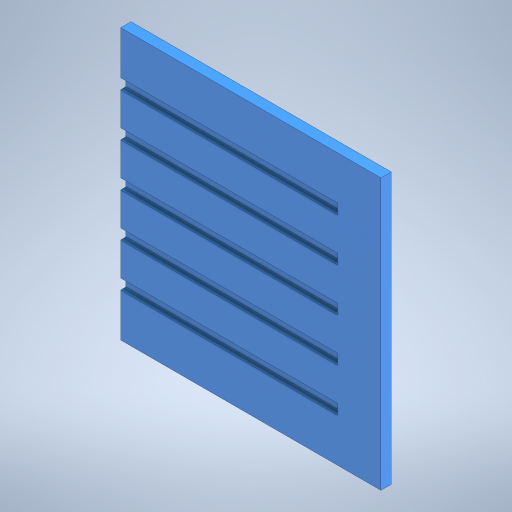
# Autodesk Inventor part: FrntBck Plate
Saved by Autodesk Inventor 2024 (Build 280153000, 153)
## iProperties
Created: 2023-10-03
Part Number: FrntBck Plate
Material: Generic
Document SubType Name: Modeling
Designer: flynf
Density: 1 g/cm^3
Appearance: Cyan
Author: flynf
Autodesk Inventor part; units mm, degrees
ref_plane "YZ Plane" through (0, 0, 0) normal (1, 0, 0) x (0, 1, 0)
ref_plane "XZ Plane" through (0, 0, 0) normal (0, 1, 0) x (-1, 0, 0)
ref_plane "XY Plane" through (0, 0, 0) normal (0, 0, 1) x (1, 0, 0)
sketch "Sketch1" plane through (0, 0, 0) normal (0, 0, 1) x (1, 0, 0)
  line L0 (0, 0) -> (279.4, 0)
  line L1 (279.4, 0) -> (279.4, 279.4)
  line L2 (279.4, 279.4) -> (0, 279.4)
  line L3 (0, 279.4) -> (0, 0)
  dimension "d0" = 279.4
  dimension "d1" = 279.4
  constraints: 8 end point, 2 parallel, 1 horizontal, 1 perpendicular
  measures "d0" distance of L0.end L1.end
  measures "d1" distance of L0.start L0.end
extrude "Extrusion1" add sketch "Sketch1" along normal blind 12.7
sketch "Sketch2" plane through (0, 0, 12.7) normal (0, 0, 1) x (1, 0, 0)
  line L0 (279.4, 0) -> (279.4, 279.4) projected
  line L1 (0, 0) -> (279.4, 0)
  line L2 (279.4, 0) -> (279.4, 12.7)
  line L3 (279.4, 12.7) -> (0, 12.7)
  line L4 (0, 12.7) -> (0, 0)
  line L5 (0, 279.4) -> (0, 0) projected
  line L6 (0, 53.34) -> (279.4, 53.34)
  line L7 (279.4, 53.34) -> (279.4, 66.04)
  line L8 (279.4, 66.04) -> (0, 66.04)
  line L9 (0, 66.04) -> (0, 53.34)
  line L10 (0, 106.68) -> (279.4, 106.68)
  line L11 (279.4, 106.68) -> (279.4, 119.38)
  line L12 (279.4, 119.38) -> (0, 119.38)
  line L13 (0, 119.38) -> (0, 106.68)
  line L14 (0, 160.02) -> (279.4, 160.02)
  line L15 (279.4, 160.02) -> (279.4, 172.72)
  line L16 (279.4, 172.72) -> (0, 172.72)
  line L17 (0, 172.72) -> (0, 160.02)
  line L18 (0, 213.36) -> (279.4, 213.36)
  line L19 (279.4, 213.36) -> (279.4, 226.06)
  line L20 (279.4, 226.06) -> (0, 226.06)
  line L21 (0, 226.06) -> (0, 213.36)
  point P0 (0, 66.04)
  point P1 (0, 119.38)
  point P2 (0, 172.72)
  point P3 (0, 226.06)
  dimension "d4" = 12.7
  dimension "d5" = 12.7
  dimension "d6" = 40.64
  dimension "d7" = 12.7
  dimension "d8" = 40.64
  dimension "d9" = 12.7
  dimension "d10" = 40.64
  dimension "d11" = 12.7
  dimension "d12" = 40.64
  constraints: 40 end point, 10 parallel, 9 point on line, 5 horizontal, 5 perpendicular
  measures "d4" distance between parallel lines of L1 L3
  measures "d5" distance between parallel lines of L8 L6
  measures "d6" distance between parallel lines of L6 L3
  measures "d7" distance between parallel lines of L12 L10
  measures "d8" distance between parallel lines of L10 L8
  measures "d9" distance between parallel lines of L16 L14
  measures "d10" distance between parallel lines of L14 L12
  measures "d11" distance between parallel lines of L20 L18
  measures "d12" distance between parallel lines of L18 L16
extrude "Extrusion2" cut sketch "Sketch2" against normal blind 6.35 contours L1 L4 L3 L0 | L6 L5 L8 L0 | L10 L5 L12 L0 | L14 L5 L16 L0 | L18 L5 L20 L0
sketch "Sketch3" plane through (279.4, 0, 0) normal (1, 0, 0) x (0, 0, -1)
  point P0 (0, 0)
sketch "Sketch4" plane through (279.4, 0, 0) normal (1, 0, 0) x (0, 0, -1)
  line L0 (-6.35, 106.68) -> (-12.7, 106.68) projected
  line L1 (-12.7, 66.04) -> (-12.7, 106.68) projected
  line L2 (-12.7, 66.04) -> (-6.35, 66.04) projected
  line L3 (-6.35, 66.04) -> (-6.35, 53.34) projected
  line L4 (-6.35, 53.34) -> (-12.7, 53.34) projected
  line L5 (-12.7, 12.7) -> (-12.7, 53.34) projected
  line L6 (-12.7, 12.7) -> (-6.35, 12.7) projected
  line L7 (-6.35, 12.7) -> (-6.35, 0) projected
  line L8 (0, 0) -> (-6.35, 0) projected
  line L9 (0, 0) -> (0, 279.4) projected
  line L10 (0, 279.4) -> (-12.7, 279.4) projected
  line L11 (-12.7, 226.06) -> (-12.7, 279.4) projected
  line L12 (-12.7, 226.06) -> (-6.35, 226.06) projected
  line L13 (-6.35, 226.06) -> (-6.35, 213.36) projected
  line L14 (-6.35, 213.36) -> (-12.7, 213.36) projected
  line L15 (-12.7, 172.72) -> (-12.7, 213.36) projected
  line L16 (-12.7, 172.72) -> (-6.35, 172.72) projected
  line L17 (-6.35, 172.72) -> (-6.35, 160.02) projected
  line L18 (-6.35, 160.02) -> (-12.7, 160.02) projected
  line L19 (-12.7, 119.38) -> (-12.7, 160.02) projected
  line L20 (-12.7, 119.38) -> (-6.35, 119.38) projected
  line L21 (-6.35, 119.38) -> (-6.35, 106.68) projected
  point P0 (0, 0)
extrude "Extrusion3" cut sketch "Sketch4" against normal blind 12.7
sketch "Sketch5" plane through (0, 0, 0) normal (0, -1, 0) x (1, 0, 0)
  line L0 (0, 0) -> (266.7, 0) projected
  line L1 (266.7, 12.7) -> (0, 12.7) projected
  line L2 (0, 0) -> (266.7, 0)
  line L3 (266.7, 0) -> (266.7, 12.7)
  line L4 (266.7, 12.7) -> (0, 12.7)
  line L5 (0, 12.7) -> (0, 0)
  constraints: 8 end point, 2 parallel, 1 horizontal, 1 perpendicular
extrude "Extrusion4" add sketch "Sketch5" along normal blind 53.34
sketch "Sketch6" plane through (266.7, 0, 0) normal (1, 0, 0) x (0, 0, -1)
  line L0 (0, 279.4) -> (0, -53.34) projected
  line L1 (-12.7, 279.4) -> (-12.7, 226.06) projected
  line L2 (0, -53.34) -> (-12.7, -53.34)
  line L3 (-12.7, -53.34) -> (-12.7, 279.4)
  line L4 (-12.7, 279.4) -> (0, 279.4)
  line L5 (0, 279.4) -> (0, -53.34)
  point P0 (0, 0)
  constraints: 8 end point, 2 parallel, 1 horizontal, 1 perpendicular
extrude "Extrusion5" add sketch "Sketch6" along normal blind 53.34
body "Solid1"
